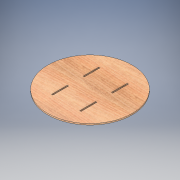
# Autodesk Inventor part: turretBasePlate
Saved by Autodesk Inventor 2018 (Build 220112000, 112)
## iProperties
Created: 2019-02-27
Part Number: turretBasePlate
Material: Generic
Document SubType Name: Modeling
Designer: snipe
Density: 1 g/cm^3
Appearance: Default
Author: snipe
Autodesk Inventor part; units mm, degrees
ref_plane "YZ Plane" through (0, 0, 0) normal (1, 0, 0) x (0, 1, 0)
ref_plane "XZ Plane" through (0, 0, 0) normal (0, 1, 0) x (-1, 0, 0)
ref_plane "XY Plane" through (0, 0, 0) normal (0, 0, 1) x (1, 0, 0)
sketch "Sketch1" plane through (0, 0, 0) normal (0, 1, 0) x (-1, 0, 0)
  circle A0 centre (0, 0) radius 203.2
  line L0 (71.4375, -38.1) -> (65.0875, -38.1)
  line L1 (65.0875, -38.1) -> (65.0875, -114.3)
  line L2 (65.0875, -114.3) -> (71.4375, -114.3)
  line L3 (71.4375, -114.3) -> (71.4375, -38.1)
  line L4 (71.4375, -38.1) -> (65.0875, -114.3) construction
  line L5 (65.0875, -38.1) -> (71.4375, -114.3) construction
  line L6 (71.4375, 114.3) -> (65.0875, 114.3)
  line L7 (65.0875, 114.3) -> (65.0875, 38.1)
  line L8 (65.0875, 38.1) -> (71.4375, 38.1)
  line L9 (71.4375, 38.1) -> (71.4375, 114.3)
  line L10 (71.4375, 114.3) -> (65.0875, 38.1) construction
  line L11 (65.0875, 114.3) -> (71.4375, 38.1) construction
  line L12 (-65.0875, -38.1) -> (-71.4375, -38.1)
  line L13 (-71.4375, -38.1) -> (-71.4375, -114.3)
  line L14 (-71.4375, -114.3) -> (-65.0875, -114.3)
  line L15 (-65.0875, -114.3) -> (-65.0875, -38.1)
  line L16 (-65.0875, -38.1) -> (-71.4375, -114.3) construction
  line L17 (-71.4375, -38.1) -> (-65.0875, -114.3) construction
  line L18 (-65.0875, 114.3) -> (-71.4375, 114.3)
  line L19 (-71.4375, 114.3) -> (-71.4375, 38.1)
  line L20 (-71.4375, 38.1) -> (-65.0875, 38.1)
  line L21 (-65.0875, 38.1) -> (-65.0875, 114.3)
  line L22 (-65.0875, 114.3) -> (-71.4375, 38.1) construction
  line L23 (-71.4375, 114.3) -> (-65.0875, 38.1) construction
  line L24 (0, -284.48) -> (0, 284.48) projected
  line L25 (-284.48, 0) -> (284.48, 0) projected
  point P0 (68.2625, -76.2)
  point P1 (68.2625, 76.2)
  point P2 (-68.2625, -76.2)
  point P3 (-68.2625, 76.2)
  dimension "d0" = 406.4
  dimension "d1" = 6.35
  dimension "d2" = 6.35
  dimension "d3" = 76.2
  dimension "d4" = 6.35
  dimension "d5" = 6.35
  dimension "d6" = 76.2
  dimension "d7" = 76.2
  dimension "d8" = 76.2
  dimension "d9" = 152.4
  dimension "d10" = 152.4
  constraints: 48 end point, 8 midpoint, 8 parallel, 4 horizontal, 4 perpendicular, 2 collinear, 1 centre point, 1 coincident, 3 other
  measures "d0" diameter of A0
  measures "d1" distance of L2.end L1.end
  measures "d2" distance of L8.end L7.end
  measures "d3" distance of L7.end L6.end
  measures "d4" distance of L14.end L13.end
  measures "d5" distance of L20.end L19.end
  measures "d6" distance of L19.end L18.end
  measures "d7" distance of L2.end L0.start
  measures "d8" distance of L12.end L13.end
  measures "d9" distance of point (68.263, 76.2) point (68.263, -76.2)
  measures "d10" distance of point (-68.262, 76.2) point (-68.262, -76.2)
extrude "Extrusion1" add sketch "Sketch1" along normal blind 6.35
body "Solid1"
